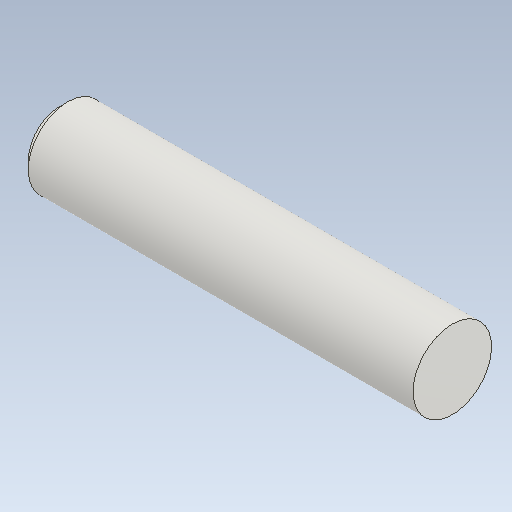
# Autodesk Inventor part: Welle
Saved by Autodesk Inventor 2021 (Build 250183000, 183)
## iProperties
CustomPartVersion: 1
Created: 2021-01-23
Part Number: Welle
Material: Steel
Document SubType Name: Modeling
Designer: Jaro Machnow
Density: 1 g/cm^3
Appearance: Steel
Length: 25,000 mm
Author: Jaro Machnow
Autodesk Inventor part; units mm, degrees
ref_plane "Startebene" through (0, 0, 0) normal (1, 0, 0) x (0, 1, 0)
ref_plane "XZ Plane" through (0, 0, 0) normal (0, 1, 0) x (-1, 0, 0)
ref_plane "XY Plane" through (0, 0, 0) normal (0, 0, 1) x (1, 0, 0)
sketch "Hauptskizze" plane through (0, 0, 0) normal (0, 0, 1) x (1, 0, 0)
  line L0 (0, 0) -> (25, 0)
  line L1 (0, 0) -> (0, 2.5)
  line L2 (25, 2.5) -> (25, 0)
  line L3 (0, 2.5) -> (25, 2.5)
  dimension "d3" = 5
  constraints: 8 end point, 2 vertical, 1 horizontal
  measures "d3" diameter of L3 L0
revolve "Umdrehung1" add sketch "Hauptskizze" angle 360 about axis through (0, 0, 0) along (1, 0, 0)
chamfer "Fase2" distance 0.5 angle 45 1 edges at (0, -2.5, 0) measured on face at (0.5, -2.5, 0)
equation "\"Length\" = 25"
